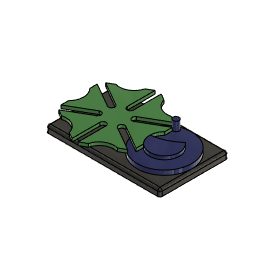
Fulg_rotit (Autodesk Fusion 360 design; units mm, degrees)
Autodesk Fusion 360 part; units mm, degrees
sketch "Base" plane through (0, 0, 0) normal (0, 0, 1) x (1, 0, 0) in component "Base"
  line L0 (-25, -15) -> (-25, 15)
  line L1 (-25, 15) -> (25, 15)
  line L2 (25, 15) -> (25, -15)
  line L3 (25, -15) -> (-25, -15)
  constraint vertical L0
  constraint perpendicular L0 L1
  constraint perpendicular L1 L2
  constraint perpendicular L0 L3
extrude "Extrude1" add sketch "Base" along normal blind 3 makes body 1 in component "Base"
fillet "Fillet1" radius 1 1 edges at (-25, 0, 3) on bodies 1 in component "Base"
fillet "Fillet2" radius 1 3 edges at (-25, -15, 1) (-24.7071, -15, 2.7071) (0.5, -15, 3) on bodies 1 in component "Base"
fillet "Fillet3" radius 1 3 edges at (25, -15, 1) (25, -14.7071, 2.7071) (25, 0.5, 3) on bodies 1 in component "Base"
fillet "Fillet4" radius 1 5 edges at (25, 15, 1) (24.7071, 15, 2.7071) (0, 15, 3) (-24.7071, 15, 2.7071) (-25, 15, 1) on bodies 1 in component "Base"
sketch "Cerc" plane through (0, 0, 3) normal (0, 0, 1) x (-1, 0, 0) in component "Cerc"
  line L0 (-24, -14) -> (24, -14)
  line L1 (24, -14) -> (24, 14)
  line L2 (24, 14) -> (-24, 14)
  line L3 (-24, 14) -> (-24, -14)
  circle A0 centre (-12, 0) radius 12
  circle A1 centre (-12, 0) radius 6.5
  constraint tangent L3 A0
  constraint concentric A0 A1
extrude "Extrude1'" add sketch "Cerc" along normal blind 2 separate body contours A0 makes body 2 in component "Cerc"
extrude "Extrude2" add sketch "Cerc" along normal blind 3.5 contours A1 bodies 2 in component "Cerc"
sketch "Fulg" plane through (0, 0, 3) normal (0, 0, 1) x (-1, 0, 0) in component "Fulg"
  line L0 (-24, 14) -> (-24, -14)
  arc A0 (-7.4545, -4.6463) -> (-7.4545, 4.6463) centre (-12, 0) ccw
  line L1 (-7.4545, 7.9412) -> (-7.4545, 4.6463)
  line L2 (-7.4545, -4.6463) -> (-7.4545, -7.9412)
  line L3 (23.5, 0) -> (24, 0)
  line L4 (25.4545, -7.9412) -> (25.4545, -4.6463)
  line L5 (25.4545, 4.6463) -> (25.4545, 7.9412)
  arc A1 (25.4545, 4.6463) -> (25.4545, -4.6463) centre (30, 0) ccw
  arc A2 (21.2511, -11.9268) -> (13.2034, -16.5732) centre (19.5, -18.1865) ccw
  line L6 (10.35, -18.2206) -> (13.2034, -16.5732)
  line L7 (21.2511, -11.9268) -> (24.1045, -10.2794)
  line L8 (24.1045, 10.2794) -> (21.2511, 11.9268)
  line L9 (13.2034, 16.5732) -> (10.35, 18.2206)
  arc A3 (13.2034, 16.5732) -> (21.2511, 11.9268) centre (19.5, 18.1865) ccw
  arc A4 (4.7966, -16.5732) -> (-3.2511, -11.9268) centre (-1.5, -18.1865) ccw
  line L10 (-6.1045, -10.2794) -> (-3.2511, -11.9268)
  line L11 (4.7966, -16.5732) -> (7.65, -18.2206)
  arc A5 (-3.2511, 11.9268) -> (4.7966, 16.5732) centre (-1.5, 18.1865) ccw
  line L12 (-3.2511, 11.9268) -> (-6.1045, 10.2794)
  line L13 (7.65, 18.2206) -> (4.7966, 16.5732)
  line L14 (13.5212, -4.1691) -> (24.1045, -10.2794)
  line L15 (14.8712, -1.8309) -> (25.4545, -7.9412)
  arc A6 (14.8712, -1.8309) -> (13.5212, -4.1691) centre (14.1962, -3) ccw
  line L16 (7.65, -6) -> (7.65, -18.2206)
  line L17 (10.35, -6) -> (10.35, -18.2206)
  arc A7 (10.35, -6) -> (7.65, -6) centre (9, -6) ccw
  line L18 (13.5212, 4.1691) -> (24.1045, 10.2794)
  line L19 (14.8712, 1.8309) -> (25.4545, 7.9412)
  line L20 (10.35, 6) -> (10.35, 18.2206)
  line L21 (7.65, 6) -> (7.65, 18.2206)
  line L22 (3.1288, 1.8309) -> (-7.4545, 7.9412)
  line L23 (4.4788, 4.1691) -> (-6.1045, 10.2794)
  line L24 (4.4788, -4.1691) -> (-6.1045, -10.2794)
  line L25 (3.1288, -1.8309) -> (-7.4545, -7.9412)
  arc A8 (4.4788, -4.1691) -> (3.1288, -1.8309) centre (3.8038, -3) ccw
  arc A9 (3.1288, 1.8309) -> (4.4788, 4.1691) centre (3.8038, 3) ccw
  arc A10 (7.65, 6) -> (10.35, 6) centre (9, 6) ccw
  arc A11 (13.5212, 4.1691) -> (14.8712, 1.8309) centre (14.1962, 3) ccw
  point P0 (9, 0)
  constraint coincident A0.start L1
  constraint collinear L1 L2
  constraint collinear L4 L5
  constraint coincident A2.start L6
  constraint collinear L6 L7
  constraint collinear L8 L9
  constraint coincident A4.start L10
  constraint collinear L10 L11
  constraint coincident A5.start L13
  constraint collinear L12 L13
  constraint coincident A1 L3.start
  constraint tangent L14 A6
  constraint tangent L15 A6
  constraint tangent L16 A7
  constraint tangent L17 A7
  constraint tangent L18 A11
  constraint tangent L19 A11
  constraint tangent L20 A10
  constraint tangent L21 A10
  constraint tangent L22 A9
  constraint tangent L23 A9
  constraint tangent L24 A8
  constraint tangent L25 A8
extrude "Extrude1''" add sketch "Fulg" along normal blind 1.4 separate body makes body 3 in component "Fulg"
move_body "Move1" bodies 3 to x (1, 0, 0) y (0, 1, 0) z (0, 0, 1) at (0, 0, 2.1) in component "Fulg"
sketch "Fulg_base1" plane through (0, 0, 3) normal (0, 0, 1) x (-1, 0, 0) in component "Fulg"
  line L0 (-24, -14) -> (24, -14)
  line L1 (24, -14) -> (24, 14)
  line L2 (24, 14) -> (-24, 14)
  line L3 (-24, 14) -> (-24, -14)
  circle A0 centre (9, 0) radius 2
extrude "Extrude2'" add sketch "Fulg_base1" along normal blind 2.1 contours A0 bodies 3 in component "Fulg"
sketch "Fulg_base2" plane through (0, 0, 0) normal (0, 0, -1) x (1, 0, 0) in component "Fulg"
  arc A0 (24, -15) -> (25, -14) centre (24, -14) ccw
  line L0 (25, -14) -> (25, 14)
  arc A1 (25, 14) -> (24, 15) centre (24, 14) ccw
  line L1 (24, 15) -> (-24, 15)
  arc A2 (-24, 15) -> (-25, 14) centre (-24, 14) ccw
  line L2 (-25, 14) -> (-25, -14)
  arc A3 (-25, -14) -> (-24, -15) centre (-24, -14) ccw
  line L3 (-24, -15) -> (24, -15)
  circle A4 centre (-9, 0) radius 0.6
extrude "Extrude3" add sketch "Fulg_base2" against normal blind 3 contours A4 bodies 3 in component "Fulg"
extrude "Extrude2''" cut sketch "Fulg_base2" against normal blind 3 contours A4 bodies 1 in component "Base"
sketch "Cerc_base" plane through (0, 0, 0) normal (0, 0, -1) x (1, 0, 0) in component "Cerc"
  circle A0 centre (-9, 0) radius 0.6
  arc A1 (24, -15) -> (25, -14) centre (24, -14) ccw
  line L0 (25, -14) -> (25, 14)
  arc A2 (25, 14) -> (24, 15) centre (24, 14) ccw
  line L1 (24, 15) -> (-24, 15)
  arc A3 (-24, 15) -> (-25, 14) centre (-24, 14) ccw
  line L2 (-25, 14) -> (-25, -14)
  arc A4 (-25, -14) -> (-24, -15) centre (-24, -14) ccw
  line L3 (-24, -15) -> (24, -15)
  circle A5 centre (12, 0) radius 2.3
extrude "Extrude3'" add sketch "Cerc_base" against normal blind 3 contours A5 bodies 2 in component "Cerc"
extrude "Extrude3''" cut sketch "Cerc_base" against normal blind 3 contours A5 bodies 1 in component "Base"
sketch "Misca_fulg" plane through (0, 0, 5) normal (0, 0, 1) x (-1, 0, 0) in component "Cerc"
  circle A0 centre (-12, 0) radius 6.5
  circle A1 centre (-12, 0) radius 12
  circle A2 centre (-6.7788, -9.11) radius 1.325
  line L0 (-7.4525, -7.9425) -> (-7.441, -7.9624)
  line L1 (-6.1165, -10.2576) -> (-6.105, -10.2775)
  line L2 (-12, 0) -> (-1.5, 0)
  circle A3 centre (-1.5, 0) radius 1.325
  dimension "d49" = 2.65
  dimension "d56" = 10.5
  dimension "d57" = 2.65
  constraint coincident A2 L0.end
  constraint coincident A2 L1.start
  constraint collinear L0 L1
  constraint coincident A2.centre L0
  constraint coincident A0.centre A1.centre
  constraint horizontal L2
  constraint coincident L2.end A3.centre
  measures "d49" diameter of A2
  measures "d56" distance of A0.centre L2.end
  measures "d57" diameter of A3
extrude "Extrude4" add sketch "Misca_fulg" along normal blind 1.5 contours A2 bodies 2 in component "Cerc"
sketch "Spatiu_fulg" plane through (0, 0, 6.5) normal (0, 0, 1) x (-1, 0, 0) in component "Cerc"
  circle A0 centre (-12, 0) radius 6.5
  arc A1 (-9.0893, -5.8119) -> (-9.0893, 5.8119) centre (-12, 0) ccw
  arc A2 (-9.0893, 5.8119) -> (-9.0893, -5.8119) centre (9, 0) ccw
  constraint concentric A0 A1
extrude "Extrude6" cut sketch "Spatiu_fulg" against normal blind 1.5 contours A0 A1 A2 bodies 2 in component "Cerc"
extrude "Extrude5" cut sketch "Spatiu_fulg" against normal blind 1.5 contours A0 A1 A2 bodies 2 in component "Cerc"
extrude "Extrude7" cut sketch "Misca_fulg" along normal blind 3 contours A2 bodies 2 in component "Cerc"
extrude "Extrude8" add sketch "Misca_fulg" along normal blind 1.5 contours A3 bodies 2 in component "Cerc"
move_body "Move1'" bodies 2 to x (0.422618, -0.906308, 0) y (0.906308, 0.422618, 0) z (0, 0, 1) at (6.9286, 10.8757, 0) in component "Cerc"
extrude "Extrude9" add 1 faces at (7.3456, 9.724, 6.5) along direction (0, 0, 1) blind 2.5 on bodies 2 bodies 2 in component "Cerc"
component "Base" placed x (1, 0, 0) y (0, 1, 0) z (0, 0, 1) at (0, 0, 0)
component "Fulg" placed x (1, 0, 0) y (0, 1, 0) z (0, 0, 1) at (0, 0, 0)
component "Cerc" placed x (1, 0, 0) y (0, 1, 0) z (0, 0, 1) at (0, 0, 0)
named bodies: "Base", "Fulg"
